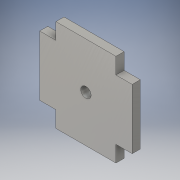
# Autodesk Inventor part: MotorRear
Saved by Autodesk Inventor 2016 (Build 200138000, 138)
## iProperties
Created: 2016-11-29
Part Number: MotorRear
Material: Generic
Document SubType Name: Modeling
Designer: Evan Phil George
Density: 1 g/cm^3
Appearance: Default
Author: Evan Phil George
Autodesk Inventor part; units mm, degrees
ref_plane "YZ Plane" through (0, 0, 0) normal (1, 0, 0) x (0, 1, 0)
ref_plane "XZ Plane" through (0, 0, 0) normal (0, 1, 0) x (-1, 0, 0)
ref_plane "XY Plane" through (0, 0, 0) normal (0, 0, 1) x (1, 0, 0)
sketch "Sketch3" plane through (0, 0, 0) normal (0, 0, 1) x (1, 0, 0)
  line L0 (-28.5, 28.5) -> (28.5, 28.5)
  line L1 (28.5, 28.5) -> (28.5, -28.5)
  line L2 (28.5, -28.5) -> (-28.5, -28.5)
  line L3 (-28.5, -28.5) -> (-28.5, 28.5)
  circle A0 centre (0, 0) radius 3.2
  line L4 (-18.5, 28.5) -> (-18.5, 18.5)
  line L5 (-18.5, 18.5) -> (-28.5, 18.5)
  line L6 (18.5, 28.5) -> (18.5, 18.5)
  line L7 (18.5, 18.5) -> (28.5, 18.5)
  line L8 (28.5, -18.5) -> (18.5, -18.5)
  line L9 (18.5, -18.5) -> (18.5, -28.5)
  line L10 (-18.5, -28.5) -> (-18.5, -18.5)
  line L11 (-18.5, -18.5) -> (-28.5, -18.5)
  line L12 (-18.5, 28.5) -> (18.5, 28.5)
  line L13 (28.5, 18.5) -> (28.5, -18.5)
  line L14 (18.5, -28.5) -> (-18.5, -28.5)
  line L15 (-28.5, -18.5) -> (-28.5, 18.5)
  dimension "d15" = 57
  dimension "d16" = 57
  dimension "d17" = 28.5
  dimension "d18" = 28.5
  dimension "d19" = 6.4
  dimension "d20" = 10
  dimension "d21" = 10
  dimension "d22" = 10
  dimension "d23" = 10
  dimension "d24" = 10
  dimension "d25" = 10
  dimension "d26" = 10
  dimension "d27" = 10
  constraints: 32 end point, 8 point on line, 6 perpendicular, 3 collinear, 3 vertical, 2 horizontal, 2 parallel, 1 centre point, 1 coincident
  measures "d15" distance of L0.start L0.end
  measures "d16" distance of L0.end L1.end
  measures "d17" distance from line of point (0, 0) L0
  measures "d18" distance from line of point (0, 0) L1
  measures "d19" diameter of A0
  measures "d20" distance of L4.end L5.end
  measures "d21" distance of L4.start L4.end
  measures "d22" distance of L6.start L6.end
  measures "d23" distance of L6.end L7.end
  measures "d24" distance of L8.start L8.end
  measures "d25" distance of L8.end L9.end
  measures "d26" distance of L10.end L11.end
  measures "d27" distance of L10.start L10.end
extrude "Extrusion2" add sketch "Sketch3" along normal blind 5 contours L0 L6 L7 L1 L8 L9 L2 L10 L11 L3 L5 L4
body "Solid2"
